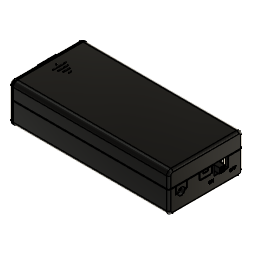
18650_2S (Autodesk Fusion 360 design; units mm, degrees)
Autodesk Fusion 360 part; units mm, degrees
note: some values were not read from the file. Set by a fixed rule: which face or edge a step refers to.
sketch "Sketch1" plane through (0, 0, 0) normal (0, 0, 1) x (1, 0, 0)
  line L0 (46, -21.4) -> (-46, -21.4)
  line L1 (-46, -21.4) -> (-46, 21.4)
  line L2 (-46, 21.4) -> (46, 21.4)
  line L3 (46, 21.4) -> (46, -21.4)
  line L4 (46, -21.4) -> (-46, 21.4) construction
  line L5 (-46, -21.4) -> (46, 21.4) construction
  dimension "d1" = 92
  dimension "d2" = 42.8
  constraint horizontal L0
  constraint perpendicular L0 L1
  constraint parallel L0 L2
  constraint parallel L1 L3
  constraint coincident L4 origin
  constraint coincident L5 origin
  measures "d1" distance of L1.end L2.end
  measures "d2" distance of L0.end L1.end
extrude "Extrude1" add sketch "Sketch1" along normal blind 22.5
sketch "Sketch2" plane through (-46, 0, 0) normal (-1, 0, 0) x (0, -1, 0)
  line L0 (-21.4, 0) -> (21.4, 0)
  line L1 (21.4, 0) -> (21.4, 22.5)
  line L2 (21.4, 22.5) -> (-21.4, 22.5)
  line L3 (-21.4, 22.5) -> (-21.4, 0)
  line L4 (-5, 21.5) -> (5, 21.5)
  line L5 (5, 21.5) -> (5, 18.5)
  line L6 (5, 18.5) -> (-5, 18.5)
  line L7 (-5, 18.5) -> (-5, 21.5)
  dimension "d5" = 10
  dimension "d6" = 3
  dimension "d7" = 16.4
  dimension "d8" = 1
  constraint horizontal L4
  constraint vertical L5
  constraint horizontal L6
  constraint vertical L7
  measures "d5" distance of L4.start L4.end
  measures "d6" distance of L4.start L6.end
  measures "d7" distance of L3 L7
  measures "d8" distance of L2 L4
extrude "Extrude2" cut sketch "Sketch2" against normal blind 2 contours L4 L5 L6 L7
sketch "Sketch3" plane through (-44, 0, 0) normal (-1, 0, 0) x (0, -1, 0)
  line L0 (-5, 18.5) -> (5, 18.5)
  line L1 (5, 18.5) -> (5, 21.5)
  line L2 (5, 21.5) -> (-5, 21.5)
  line L3 (-5, 21.5) -> (-5, 18.5)
  line L4 (-4.25, 21) -> (4.25, 21)
  line L5 (4.25, 21) -> (4.25, 19.5)
  line L6 (4.25, 19.5) -> (-4.25, 19.5)
  line L7 (-4.25, 19.5) -> (-4.25, 21)
  dimension "d11" = 8.5
  dimension "d12" = 1.5
  dimension "d13" = 1
  dimension "d14" = 0.75
  constraint horizontal L4
  constraint vertical L5
  constraint horizontal L6
  constraint vertical L7
  measures "d11" distance of L4.start L4.end
  measures "d12" distance of L4.start L6.end
  measures "d13" distance of L0 L6
  measures "d14" distance of L3 L7
extrude "Extrude3" add sketch "Sketch3" along normal blind 2 contours L4 L5 L6 L7
sketch "Sketch4" plane through (0, 0, 22.5) normal (0, 0, 1) x (-1, 0, 0)
  line L0 (-46, -21.4) -> (46, -21.4)
  line L1 (46, -21.4) -> (46, 21.4)
  line L2 (46, 21.4) -> (-46, 21.4)
  line L3 (-46, 21.4) -> (-46, -21.4)
  line L4 (43.75, 21.4) -> (44, 21.4)
  line L5 (44, 21.4) -> (44, -21.4)
  line L6 (44, -21.4) -> (43.75, -21.4)
  line L7 (43.75, -21.4) -> (43.75, 21.4)
  dimension "d17" = 0.25
  dimension "d18" = 2
  constraint horizontal L4
  constraint vertical L5
  constraint horizontal L6
  constraint vertical L7
  constraint coincident L0 L5.end
  constraint coincident L2 L4.start
  measures "d17" distance of L4.start L4.end
  measures "d18" distance of L1 L5
extrude "Extrude4" cut sketch "Sketch4" against normal blind 0.25 contours L0 L2 L4 L5 L6 L7
sketch "Sketch5" plane through (0, 21.4, 0) normal (0, 1, 0) x (-1, 0, 0)
  line L0 (44, 22.5) -> (44, 22.25)
  line L1 (44, 22.25) -> (43.75, 22.25)
  line L2 (43.75, 22.25) -> (43.75, 22.5)
  line L3 (43.75, 22.5) -> (-46, 22.5)
  line L4 (-46, 22.5) -> (-46, 0)
  line L5 (-46, 0) -> (46, 0)
  line L6 (46, 0) -> (46, 22.5)
  line L7 (46, 22.5) -> (44, 22.5)
  line L8 (43.75, 22.25) -> (44, 22.25)
  line L9 (44, 22.25) -> (44, 0)
  line L10 (44, 0) -> (43.75, 0)
  line L11 (43.75, 0) -> (43.75, 22.25)
  dimension "d21" = 0.25
  constraint horizontal L8
  constraint vertical L9
  constraint horizontal L10
  constraint vertical L11
  constraint coincident L5 L9.end
  constraint coincident L1.end L2.start
  measures "d4" distance of L1.end L0.end
extrude "Extrude5" cut sketch "Sketch5" against normal blind 0.25 contours L1 L5 L8 L9 L10 L11
mirror "Mirror1" about plane through (0, 0, 0) normal (0, 1, 0) of "Extrude5"
sketch "Sketch6" plane through (0, 0, 0) normal (0, 0, -1) x (1, 0, 0)
  line L0 (-44, 21.15) -> (-44, 21.4)
  line L1 (-44, 21.4) -> (-46, 21.4)
  line L2 (-46, 21.4) -> (-46, -21.4)
  line L3 (-46, -21.4) -> (-44, -21.4)
  line L4 (-44, -21.4) -> (-44, -21.15)
  line L5 (-44, -21.15) -> (-43.75, -21.15)
  line L6 (-43.75, -21.15) -> (-43.75, -21.4)
  line L7 (-43.75, -21.4) -> (46, -21.4)
  line L8 (46, -21.4) -> (46, 21.4)
  line L9 (46, 21.4) -> (-43.75, 21.4)
  line L10 (-43.75, 21.4) -> (-43.75, 21.15)
  line L11 (-43.75, 21.15) -> (-44, 21.15)
  line L12 (-44, 21.15) -> (-43.75, 21.15)
  line L13 (-43.75, 21.15) -> (-43.75, -21.15)
  line L14 (-43.75, -21.15) -> (-44, -21.15)
  line L15 (-44, -21.15) -> (-44, 21.15)
  constraint horizontal L12
  constraint vertical L13
  constraint horizontal L14
  constraint vertical L15
  constraint coincident L5.end L6.start
  constraint coincident L0.start L11.end
extrude "Extrude6" cut sketch "Sketch6" against normal blind 0.25 contours L5 L11 L12 L13 L14 L15
sketch "Sketch7" plane through (0, 21.4, 0) normal (0, 1, 0) x (-1, 0, 0)
  line L0 (43.75, 0) -> (43.75, 22.5)
  line L1 (43.75, 22.5) -> (-46, 22.5)
  line L2 (-46, 22.5) -> (-46, 0)
  line L3 (-46, 0) -> (43.75, 0)
  line L4 (43.75, 13.45) -> (-46, 13.45)
  line L5 (-46, 13.45) -> (-46, 13.2)
  line L6 (-46, 13.2) -> (43.75, 13.2)
  line L7 (43.75, 13.2) -> (43.75, 13.45)
  dimension "d28" = 0.25
  dimension "d29" = 13.2
  constraint horizontal L4
  constraint vertical L5
  constraint horizontal L6
  constraint vertical L7
  constraint coincident L2 L5.end
  constraint coincident L0 L4.start
  measures "d4" distance of L4.start L6.end
  measures "d29" distance of L3 L6
extrude "Extrude7" cut sketch "Sketch7" against normal blind 0.25 contours L0 L2 L4 L5 L6 L7
mirror "Mirror2" about plane through (0, 0, 0) normal (0, 1, 0) of "Extrude7"
sketch "Sketch8" plane through (46, 0, 0) normal (1, 0, 0) x (0, 1, 0)
  line L0 (-21.4, 13.45) -> (-21.15, 13.45)
  line L1 (-21.15, 13.45) -> (-21.15, 13.2)
  line L2 (-21.15, 13.2) -> (-21.4, 13.2)
  line L3 (-21.4, 13.2) -> (-21.4, 0)
  line L4 (-21.4, 0) -> (21.4, 0)
  line L5 (21.4, 0) -> (21.4, 13.2)
  line L6 (21.4, 13.2) -> (21.15, 13.2)
  line L7 (21.15, 13.2) -> (21.15, 13.45)
  line L8 (21.15, 13.45) -> (21.4, 13.45)
  line L9 (21.4, 13.45) -> (21.4, 22.5)
  line L10 (21.4, 22.5) -> (-21.4, 22.5)
  line L11 (-21.4, 22.5) -> (-21.4, 13.45)
  line L12 (-21.15, 13.45) -> (21.15, 13.45)
  line L13 (21.15, 13.45) -> (21.15, 13.2)
  line L14 (21.15, 13.2) -> (-21.15, 13.2)
  line L15 (-21.15, 13.2) -> (-21.15, 13.45)
  line L16 (-3.75, 13.2) -> (3.75, 13.2)
  line L17 (3.75, 13.2) -> (3.75, 10.2)
  line L18 (2.75, 9.2) -> (-2.75, 9.2)
  line L19 (-3.75, 10.2) -> (-3.75, 13.2)
  line L20 (-2.75, 9.45) -> (2.75, 9.45)
  line L21 (-3.5, 13.2) -> (-3.5, 10.2)
  line L22 (3.5, 13.2) -> (3.5, 10.2)
  line L23 (-1.5, 13.2) -> (1.5, 13.2)
  line L24 (1.5, 13.2) -> (1.5, 11.7)
  line L25 (1.5, 11.7) -> (-1.5, 11.7)
  line L26 (-1.5, 11.7) -> (-1.5, 13.2)
  line L27 (-1.3, 13.2) -> (1.3, 13.2)
  line L28 (1.3, 13.2) -> (1.3, 11.9)
  line L29 (1.3, 11.9) -> (-1.3, 11.9)
  line L30 (-1.3, 11.9) -> (-1.3, 13.2)
  arc A0 (-3.5, 10.2) -> (-2.75, 9.45) centre (-2.75, 10.2) ccw
  arc A1 (2.75, 9.45) -> (3.5, 10.2) centre (2.75, 10.2) ccw
  arc A2 (-3.75, 10.2) -> (-2.75, 9.2) centre (-2.75, 10.2) ccw
  arc A3 (2.75, 9.2) -> (3.75, 10.2) centre (2.75, 10.2) ccw
  line L31 (-17.4, 13.2) -> (-10.8, 13.2)
  line L32 (-10.8, 13.2) -> (-10.8, 9.2)
  line L33 (-10.8, 9.2) -> (-17.4, 9.2)
  line L34 (-17.4, 9.2) -> (-17.4, 13.2)
  line L35 (-17.4, 9.7) -> (-10.8, 9.7)
  line L36 (-17.15, 13.2) -> (-17.15, 9.7)
  line L37 (-11.05, 13.2) -> (-11.05, 9.7)
  circle A4 centre (-14.1, 9.2) radius 2
  line L38 (4.9, 13.45) -> (12.9, 13.45)
  line L39 (12.9, 13.45) -> (12.9, 7.45)
  line L40 (12.9, 7.45) -> (4.9, 7.45)
  line L41 (4.9, 7.45) -> (4.9, 13.45)
  point P0 (-3.75, 9.2)
  dimension "d34" = 7.5
  dimension "d35" = 4
  dimension "d36" = 17.65
  dimension "d37" = 0.25
  dimension "d38" = 0.25
  dimension "d39" = 0.25
  dimension "d40" = 3
  dimension "d41" = 1.5
  dimension "d42" = 2
  dimension "d43" = 2.6
  dimension "d44" = 1.3
  dimension "d45" = 0.2
  dimension "d46" = 0.75
  dimension "d47" = 1
  dimension "d48" = 6.6
  dimension "d49" = 4
  dimension "d50" = 4
  dimension "d51" = 0.5
  dimension "d52" = 0.25
  dimension "d53" = 0.25
  dimension "d54" = 4
  dimension "d55" = 8
  dimension "d56" = 6
  dimension "d57" = 8.5
  constraint horizontal L12
  constraint vertical L13
  constraint horizontal L14
  constraint vertical L15
  constraint coincident L6.end L7.start
  constraint coincident L0.end L1.start
  constraint horizontal L16
  constraint vertical L17
  constraint horizontal L18
  constraint vertical L19
  constraint coincident L14 L16.start
  constraint perpendicular L17 L20
  constraint coincident L16 L21.start
  constraint perpendicular L20 L21
  constraint coincident L16 L22.start
  constraint perpendicular L20 L22
  constraint horizontal L23
  constraint vertical L24
  constraint horizontal L25
  constraint vertical L26
  constraint coincident L16 L23.start
  constraint horizontal L27
  constraint vertical L28
  constraint horizontal L29
  constraint vertical L30
  constraint coincident L23 L27.start
  constraint tangent L21 A0
  constraint tangent L20 A0
  constraint tangent L22 A1
  constraint tangent L20 A1
  constraint equal A0 A1
  constraint coincident P0 L19
  constraint coincident P0 L18
  constraint tangent L19 A2
  constraint tangent L18 A2
  constraint tangent L17 A3
  constraint tangent L18 A3
  constraint equal A2 A3
  constraint horizontal L31
  constraint vertical L32
  constraint horizontal L33
  constraint vertical L34
  constraint coincident L14 L31.start
  constraint coincident L34 L35.start
  constraint coincident L32 L35.end
  constraint perpendicular L32 L35
  constraint coincident L14 L36.start
  constraint coincident L35 L36.end
  constraint perpendicular L35 L36
  constraint coincident L14 L37.start
  constraint coincident L35 L37.end
  constraint perpendicular L35 L37
  constraint midpoint L33 A4.centre
  constraint horizontal L38
  constraint vertical L39
  constraint horizontal L40
  constraint vertical L41
  constraint coincident L12 L38.start
  measures "d34" distance of L16.start L16.end
  measures "d35" distance of L16.start P0
  measures "d36" distance of L5 L17
  measures "d37" distance of L18 L20
  measures "d38" distance of L19 L21
  measures "d39" distance of L17 L22
  measures "d40" distance of L23.start L23.end
  measures "d41" distance of L23.start L25.end
  measures "d42" distance of L22 L24
  measures "d43" distance of L27.start L27.end
  measures "d44" distance of L27.start L29.end
  measures "d45" distance of L26 L30
  measures "d46" radius of A0
  measures "d47" radius of A2
  measures "d48" distance of L31.start L31.end
  measures "d49" distance of L31.start L33.end
  measures "d50" distance of L3 L34
  measures "d51" distance of L33 L35
  measures "d52" distance of L34 L36
  measures "d53" distance of L32 L37
  measures "d54" diameter of A4
  measures "d55" distance of L38.start L38.end
  measures "d56" distance of L38.start L40.end
  measures "d57" distance of L5 L39
extrude "Extrude8" cut sketch "Sketch8" against normal blind 0.25 contours L1 L12 L14 L15 L16 L23 L27 L31 L41 | L14 L31 L34 L35 L36 | L7 L12 L13 L14 L39 | L33 L34 L35 A4 | L14 L16 L17 L18 L19 L20 L21 L22 A0 A1 A2 A3 | L14 L31 L32 L35 L37 | L32 L33 L35 A4 | L14 L16 L23 L24 L25 L26 L28 L29 L30
extrude "Extrude9" cut sketch "Sketch8" against normal blind 2 contours L12 L14 L38 L39 L41 | L14 L39 L40 L41 | L35 A4 | L33 L35 A4 | L33 A4
sketch "Sketch9" plane through (44, 0, 0) normal (1, 0, 0) x (0, 1, 0)
  line L0 (4.9, 7.45) -> (12.9, 7.45)
  line L1 (12.9, 7.45) -> (12.9, 13.45)
  line L2 (12.9, 13.45) -> (4.9, 13.45)
  line L3 (4.9, 13.45) -> (4.9, 7.45)
  line L4 (4.9, 12.95) -> (12.9, 12.95)
  line L5 (12.9, 12.95) -> (12.9, 7.95)
  line L6 (12.9, 7.95) -> (4.9, 7.95)
  line L7 (4.9, 7.95) -> (4.9, 12.95)
  line L8 (11.9, 8.95) -> (5.9, 8.95)
  line L9 (5.9, 8.95) -> (5.9, 11.95)
  line L10 (5.9, 11.95) -> (11.9, 11.95)
  line L11 (11.9, 11.95) -> (11.9, 8.95)
  line L12 (11.9, 11.95) -> (10.4, 11.95)
  line L13 (10.4, 11.95) -> (10.4, 8.95)
  line L14 (10.4, 8.95) -> (11.9, 8.95)
  line L15 (11.9, 8.95) -> (11.9, 11.95)
  line L16 (5.9, 11.95) -> (8.9, 11.95)
  line L17 (8.9, 11.95) -> (8.9, 8.95)
  line L18 (8.9, 8.95) -> (5.9, 8.95)
  line L19 (5.9, 8.95) -> (5.9, 11.95)
  dimension "d62" = 0.5
  dimension "d63" = 0.5
  dimension "d64" = 1
  dimension "d67" = 1.5
  dimension "d70" = 3
  dimension "d71" = 3
  constraint horizontal L4
  constraint vertical L5
  constraint horizontal L6
  constraint vertical L7
  constraint coincident L1 L5.end
  constraint coincident L3 L4.start
  constraint horizontal L12
  constraint vertical L13
  constraint horizontal L14
  constraint vertical L15
  constraint coincident L8 L13.end
  constraint horizontal L16
  constraint vertical L17
  constraint horizontal L18
  constraint vertical L19
  measures "d62" distance of L2 L4
  measures "d63" distance of L0 L6
  measures "d67" distance of L10.end L12.end
  measures "d70" distance of L9.end L16.end
  measures "d71" distance of L9.end L8.end
extrude "Extrude10" add sketch "Sketch9" along normal blind 0.5 contours L1 L3 L4 L5 L6 L7
extrude "Extrude11" cut sketch "Sketch9" against normal blind 1 contours L8 L10 L11 L12 L13 L14 L15
extrude "Extrude12" add sketch "Sketch9" along normal blind 4 contours L8 L9 L10 L16 L17 L18 L19
fillet "Fillet1" radius 0.4 2 edges at (43.75, 11.9, 11.95) (43.75, 11.9, 8.95)
fillet "Fillet1" radius 0.2 2 edges at (44.5, 8.9, 12.95) (44.5, 8.9, 7.95)
sketch "Sketch10" plane through (48, 0, 0) normal (1, 0, 0) x (0, 1, 0)
  line L0 (5.9, 8.95) -> (8.9, 8.95)
  line L1 (8.9, 8.95) -> (8.9, 11.95)
  line L2 (8.9, 11.95) -> (5.9, 11.95)
  line L3 (5.9, 11.95) -> (5.9, 8.95)
  line L4 (5.9, 11.95) -> (6.15, 11.95)
  line L5 (6.15, 11.95) -> (6.15, 8.95)
  line L6 (6.15, 8.95) -> (5.9, 8.95)
  line L7 (5.9, 8.95) -> (5.9, 11.95)
  dimension "d78" = 0.25
  constraint horizontal L4
  constraint vertical L5
  constraint horizontal L6
  constraint vertical L7
  constraint coincident L0 L5.end
  constraint coincident L2.end L3.start
  measures "d78" distance of L2.end L4.end
extrude "Extrude13" add sketch "Sketch10" along normal blind 0.25 contours L0 L2 L3 L4 L5 L6 L7
fillet "Fillet2" radius 0.125 2 edges at (48.25, 5.9, 10.45) (48.25, 6.15, 10.45)
pattern_linear "R-Pattern1" count 5 spacing 0.69 along (0, 1, 0) of "Extrude13", "Fillet2"
sketch "Sketch11" plane through (44, 0, 0) normal (1, 0, 0) x (0, 1, 0)
  circle A0 centre (-14.1, 9.2) radius 2
  circle A1 centre (-15.1, 9.2) radius 0.75
  circle A2 centre (-13.1, 9.2) radius 0.75
  line L0 (-14.1, 9.2) -> (-12.1, 9.2)
  line L1 (-14.1, 9.2) -> (-16.1, 9.2)
  dimension "d87" = 1.5
  dimension "d88" = 1.5
  dimension "d89" = 1
  dimension "d90" = 1
  constraint coincident A0.centre L0.start
  constraint coincident A0 L0.end
  constraint horizontal L0
  constraint coincident A0 L1.end
  constraint parallel L0 L1
  constraint coincident A1.centre L1
  constraint coincident A2.centre L0
  measures "d87" diameter of A1
  measures "d88" diameter of A2
  measures "d89" distance of A0.centre A1.centre
  measures "d90" horizontal distance of A0.centre A2.centre
extrude "Extrude14" add sketch "Sketch11" along normal blind 0.1 contours A2 L0 | A2 L0 | A1 L1 | A1 L1
fillet "Fillet3" radius 1 2 edges at (45.75, -21.15, 13.325) (45.75, 21.15, 13.325)
fillet "Fillet6" radius 2 4 edges at (-43.875, -21.15, 22.25) (-43.875, 21.15, 22.25) (-43.875, -21.15, 0.25) (-43.875, 21.15, 0.25)
fillet "Fillet4" radius 2.5 8 edges at (1.125, -21.4, 22.5) (1.125, -21.4, 0) (1.125, 21.4, 22.5) (1.125, 21.4, 0) (-45, 21.4, 22.5) (-45, 21.4, 0) (-45, -21.4, 22.5) (-45, -21.4, 0)
fillet "Fillet4" radius 1.25 10 edges at (46, 0, 22.5) (46, -21.4, 17.975) (46, -21.4, 6.6) (46, 21.4, 17.975) (46, 21.4, 6.6) (46, 0, 0) (-46, 0, 22.5) (-46, 21.4, 11.25) (-46, -21.4, 11.25) (-46, 0, 0)
fillet "Fillet7" radius 0.1 63 edges at (0.5, -21.4, 13.45) (45.6339, -21.0339, 13.45) (46, 0, 13.45) (45.6339, 21.0339, 13.45) (0.5, 21.4, 13.45) (0.5, 21.4, 13.2) (45.6339, 21.0339, 13.2) (46, 16.525, 13.2) (-43.75, 21.4, 16.725) (-43.75, 20.6678, 21.7678) (-43.75, 0, 22.5) (-43.75, -20.6678, 21.7678) (-43.75, -21.4, 16.725) (-44, 0, 0) (-44, -20.6678, 0.7322) (-44, -21.4, 11.25) (-44, -20.6678, 21.7678) (-44, 0, 22.5) (-44, 20.6678, 21.7678) (-44, 21.4, 11.25) (-44, 20.6678, 0.7322) (-43.75, -21.4, 7.85) (-43.75, -20.6678, 0.7322) (-43.75, 0, 0) (-43.75, 20.6678, 0.7322) (-43.75, 21.4, 7.85) (46, -18.775, 13.2) (45.6339, -21.0339, 13.2) (0.5, -21.4, 13.2) (46, -17.4, 11.2) (46, -16.75, 9.2) (46, -11.45, 9.2) (46, -10.8, 11.2) (46, -11.6068, 9.7) (46, -11.05, 11.45) (46, -14.1, 13.2) (46, -17.15, 11.45) (46, -14.1, 11.2) (46, -14.1, 7.2) (46, 3.75, 11.7) (46, 3.4571, 9.4929) (46, 0, 9.2) (46, -3.4571, 9.4929) (46, -3.75, 11.7) (46, -7.275, 13.2) (46, -2.5, 13.2) (46, 0, 13.2) (46, 0, 11.9) (46, -1.3, 12.55) (46, 1.3, 12.55) (46, 1.5, 12.45) (46, -3.5, 11.7) (46, -3.2803, 9.6697) (46, 0, 9.45) (46, 3.2803, 9.6697) (46, 3.5, 11.7) (46, -1.5, 12.45) (46, 0, 11.7) (46, 2.5, 13.2) (46, 4.325, 13.2) (46, 4.9, 10.325) (46, 8.9, 7.45) (46, 12.9, 10.325)
fillet "Fillet5" radius 0.4 8 edges at (-45.9747, 0, 21.5) (-46, 0, 18.5) (-46, 5, 19.875) (-45.9937, 5, 21.3756) (-46, 0, 19.5) (-46, 0, 21) (-45.9937, -5, 21.3756) (-46, -5, 19.875)
sketch "Sketch12" plane through (0, 0, 22.5) normal (0, 0, 1) x (-1, 0, 0)
  line L0 (43.65, -18.9) -> (43.65, 18.9)
  line L1 (43.65, 18.9) -> (-44.75, 18.9)
  line L2 (-44.75, 18.9) -> (-44.75, -18.9)
  line L3 (-44.75, -18.9) -> (43.65, -18.9)
  line L4 (38.15, -4) -> (38.65, -4)
  line L5 (38.65, -4) -> (38.65, 4)
  line L6 (38.65, 4) -> (38.15, 4)
  line L7 (38.15, 4) -> (38.15, -4)
  line L8 (38.15, -4) -> (38.65, 4) construction
  line L9 (38.65, -4) -> (38.15, 4) construction
  line L10 (38.4, 0) -> (22.4, 0)
  line L11 (36.15, -3) -> (36.65, -3)
  line L12 (36.65, -3) -> (36.65, 3)
  line L13 (36.65, 3) -> (36.15, 3)
  line L14 (36.15, 3) -> (36.15, -3)
  line L15 (36.15, -3) -> (36.65, 3) construction
  line L16 (36.65, -3) -> (36.15, 3) construction
  line L17 (34.15, -2) -> (34.65, -2)
  line L18 (34.65, -2) -> (34.65, 2)
  line L19 (34.65, 2) -> (34.15, 2)
  line L20 (34.15, 2) -> (34.15, -2)
  line L21 (34.15, -2) -> (34.65, 2) construction
  line L22 (34.65, -2) -> (34.15, 2) construction
  line L23 (32.15, -1) -> (32.65, -1)
  line L24 (32.65, -1) -> (32.65, 1)
  line L25 (32.65, 1) -> (32.15, 1)
  line L26 (32.15, 1) -> (32.15, -1)
  line L27 (32.15, -1) -> (32.65, 1) construction
  line L28 (32.65, -1) -> (32.15, 1) construction
  circle A0 centre (40.15, 0) radius 0.5
  point P0 (38.4, 0)
  point P1 (36.4, 0)
  point P2 (34.4, 0)
  point P3 (32.4, 0)
  dimension "d109" = 0.5
  dimension "d110" = 8
  dimension "d111" = 5
  dimension "d112" = 18.9
  dimension "d113" = 16
  dimension "d114" = 0.5
  dimension "d115" = 6
  dimension "d116" = 0.5
  dimension "d117" = 4
  dimension "d118" = 0.5
  dimension "d119" = 2
  dimension "d120" = 1.5
  dimension "d121" = 1.5
  dimension "d122" = 1.5
  dimension "d123" = 1
  dimension "d124" = 1.5
  dimension "d125" = 18.9
  constraint horizontal L4
  constraint perpendicular L4 L5
  constraint parallel L4 L6
  constraint parallel L5 L7
  constraint coincident L8 P0
  constraint coincident L9 P0
  constraint coincident P0 L10.start
  constraint perpendicular L7 L10
  constraint horizontal L11
  constraint perpendicular L11 L12
  constraint parallel L11 L13
  constraint parallel L12 L14
  constraint coincident L15 P1
  constraint coincident L16 P1
  constraint coincident L10 P1
  constraint horizontal L17
  constraint perpendicular L17 L18
  constraint parallel L17 L19
  constraint parallel L18 L20
  constraint coincident L21 P2
  constraint coincident L22 P2
  constraint coincident L10 P2
  constraint horizontal L23
  constraint perpendicular L23 L24
  constraint parallel L23 L25
  constraint parallel L24 L26
  constraint coincident L27 P3
  constraint coincident L28 P3
  constraint coincident L10 P3
  measures "d109" distance of L5.end L6.end
  measures "d110" distance of L4.end L5.end
  measures "d111" distance of L0 L5
  measures "d112" distance of L3 P0
  measures "d113" distance of P0 L10.end
  measures "d114" distance of L12.end L13.end
  measures "d115" distance of L11.end L12.end
  measures "d116" distance of L18.end L19.end
  measures "d117" distance of L17.end L18.end
  measures "d118" distance of L24.end L25.end
  measures "d119" distance of L23.end L24.end
  measures "d120" distance of L7 L12
  measures "d121" distance of L14 L18
  measures "d122" distance of L20 L24
  measures "d123" diameter of A0
  measures "d124" distance of L5 A0.centre
  measures "d125" distance of L3 A0.centre
extrude "Extrude15" add sketch "Sketch12" along normal blind 0.25 contours L4 L5 L6 L7 | L10 L11 L12 L14 | L10 L12 L13 L14 | L10 L17 L18 L20 | L10 L18 L19 L20 | L10 L23 L24 L26 | L10 L24 L25 L26 | A0
fillet "Fillet8" radius 0.25 5 faces at (-40.1107, 0.2982, 22.75) (-38.3167, -1.3333, 22.75) (-36.3167, -1, 22.75) (-34.3167, -0.6667, 22.75) (-32.3167, -0.3333, 22.75)
sketch "Sketch13" plane through (46, 0, 0) normal (1, 0, 0) x (0, 1, 0)
  line L0 (20.15, 13.1) -> (13, 13.1)
  line L1 (13, 13.1) -> (13, 7.35)
  line L2 (13, 7.35) -> (4.8, 7.35)
  line L3 (4.8, 7.35) -> (4.8, 13.1)
  line L4 (4.8, 13.1) -> (3.85, 13.1)
  line L5 (3.85, 13.1) -> (3.85, 10.2)
  arc A0 (2.75, 9.1) -> (3.85, 10.2) centre (2.75, 10.2) ccw
  line L6 (2.75, 9.1) -> (-2.75, 9.1)
  arc A1 (-3.85, 10.2) -> (-2.75, 9.1) centre (-2.75, 10.2) ccw
  line L7 (-3.85, 10.2) -> (-3.85, 13.1)
  line L8 (-3.85, 13.1) -> (-10.7, 13.1)
  line L9 (-10.7, 13.1) -> (-10.7, 9.1)
  line L10 (-10.7, 9.1) -> (-12.0024, 9.1)
  arc A2 (-16.1976, 9.1) -> (-12.0024, 9.1) centre (-14.1, 9.2) ccw
  line L11 (-16.1976, 9.1) -> (-17.5, 9.1)
  line L12 (-17.5, 9.1) -> (-17.5, 13.1)
  line L13 (-17.5, 13.1) -> (-20.15, 13.1)
  line L14 (-20.15, 13.1) -> (-20.15, 2.5)
  arc A3 (-20.15, 2.5) -> (-18.9, 1.25) centre (-18.9, 2.5) ccw
  line L15 (-18.9, 1.25) -> (18.9, 1.25)
  arc A4 (18.9, 1.25) -> (20.15, 2.5) centre (18.9, 2.5) ccw
  line L16 (20.15, 2.5) -> (20.15, 13.1)
  line L17 (0.9007, 4.066) -> (4.9007, 4.066) construction
  line L18 (4.9007, 4.066) -> (4.9007, 7.066) construction
  line L19 (4.9007, 7.066) -> (0.9007, 7.066) construction
  line L20 (0.9007, 7.066) -> (0.9007, 4.066) construction
  line L21 (13.5003, 4.2326) -> (17.5003, 4.2326) construction
  line L22 (17.5003, 4.2326) -> (17.5003, 7.2326) construction
  line L23 (17.5003, 7.2326) -> (13.5003, 7.2326) construction
  line L24 (13.5003, 7.2326) -> (13.5003, 4.2326) construction
  dimension "d130" = 1.5
  dimension "d131" = 1.5
  text T0 "ON" font "Verdana" height 1.5 align centre middle in box 4 x 3 at (0.9007, 4.066) x (1, 0) y (0, 1) spacing 1 kerned
  text T1 "OFF" font "Verdana" height 1.5 align centre middle in box 4 x 3 at (13.5003, 4.2326) x (1, 0) y (0, 1) spacing 1 kerned
extrude "Extrude16" add sketch "Sketch13" along normal blind 0.25 text T0 T1
fillet "Fillet9" radius 0.05 5 faces at (46.25, 13.7169, 5.6472) (46.25, 15.3497, 5.7233) (46.25, 16.5354, 5.7233) (46.25, 1.6169, 5.4806) (46.25, 4.2655, 5.4077)
named bodies: "18650_2S"
